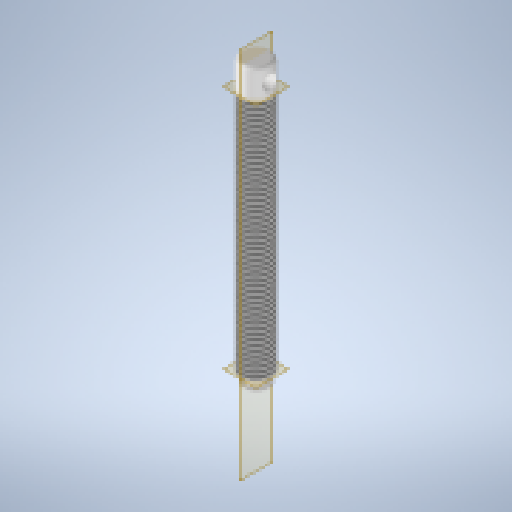
# Autodesk Inventor part: clampScrew
Saved by Autodesk Inventor 2024.2 (Build 282272000, 272)
## iProperties
Created: 2024-05-25
Part Number: clampScrew
Material: Generic
Document SubType Name: Modeling
Designer: user
Density: 1 g/cm^3
Appearance: Default
Author: user
Autodesk Inventor part; units mm, degrees
ref_plane "YZ Plane" through (0, 0, 0) normal (1, 0, 0) x (0, 1, 0)
ref_plane "XY Plane" through (0, 0, 0) normal (0, 0, 1) x (1, 0, 0)
sketch "Sketch1" plane through (0, 0, 0) normal (0, 1, 0) x (-1, 0, 0)
  circle A0 centre (0, 0) radius 4
  circle A1 centre (0, 0) radius 2.25
  dimension "d0" = 8
  dimension "d3" = 4.5
  constraints: 2 centre point, 2 coincident
  measures "d0" diameter of A0
  measures "d3" diameter of A1
extrude "Extrusion1" add sketch "Sketch1" along normal blind 80 contours A0 | A1
extrude "Extrusion2" cut sketch "Sketch1" along normal blind 7
sketch "Sketch2" plane through (0, 0, 0) normal (1, 0, 0) x (0, 1, 0)
  line L0 (80, -4) -> (80, 4) projected
  circle A0 centre (76, 0) radius 2
  point P0 (0, 0)
  dimension "d6" = 4
  dimension "d7" = 4
  constraints: 1 centre point, 1 coincident
  measures "d6" distance from line of L0 point (76, 0)
  measures "d7" diameter of A0
extrude "Extrusion3" cut sketch "Sketch2" along normal through all both and the other way through all
thread "Thread1" size "M8x1.25" class "6g" standard "ANSI Metric M Profile" length 65
fillet "Fillet1" radius 1 2 edges at (4, 80, 0) (2.25, 0, 0)
ref_plane "Work Plane1" through (0, 73, 0) normal (0, 1, 0) x (-1, 0, 0)
ref_plane "Work Plane2" through (0, 7, 0) normal (0, 1, 0) x (-1, 0, 0)
extrude "Extrusion4" cut sketch "Sketch1" along normal blind 4 contours A1
sketch "Sketch3" plane through (0, 4, 0) normal (0, -1, 0) x (1, 0, 0)
  circle A0 centre (0, -0.1147) radius 3.4149
  point P0 (0, 0)
  constraints: 1 centre point
extrude "Extrusion5" add sketch "Sketch3" against normal blind 0.35
fillet "Fillet3" radius 0.2 1 edges at (-3.4149, 4, -0.1147)
body "Solid1"
